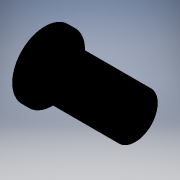
# Autodesk Inventor part: HFROLL5_a
Saved by Autodesk Inventor 2017.3 (Build 213256000, 256)
## iProperties
Part Number: HFROLL5_a
Material: Generic
Catalog Web Link: www.cadenas.de
Description: HFROLL, HFROLLM_ac-Rollers for Aluminum Frames
Vendor: MISUMI
Document SubType Name: Modeling
Designer: partserver
Manufacturer: MISUMI
Mass: 0.70535 g
Surface Area: 10.8347 cm^2
Volume: 0.70535 cm^3
Density: 1 g/cm^3
Appearance: PSOLRGB-0-0-0
Category: PARTsolutions
Company: MISUMI
Title: HFROLL5
Author: Cadenas PARTsolutions
Comments: Rollers for Aluminum Frames
PSOL_IDENT_0: {$CADENAS_DATA\23d-libs\misumi\metric\39_accessories_for_al_extrusions\hfroll\hfroll_ac.prj},173 {VT
PSOL_IDENT_1: YP=3D},{NB=HFROLL5_a},{LINA=HFROLL5},{NN=HFROLL, HFROLLM_ac},{DATE=30.03.2018 07:06:35},{GEOMDATE=10
PSOL_IDENT_2: .06.2016 08:24:00},{VERSION=},{LINEID=10},{WBVAR=MATAC},{WBNUMERIC=}  {NB=HFROLL5_a},{LINA=HFROLL5},
PSOL_IDENT_3: {KT=DUMMY},{PN=HFROLL5},{MATAC=HFROLL},{MATR=Nylon 6},{TYPE=HFROLL},{NO=5},{CFSW=6},{CFT=20-40 Sq.},
PSOL_IDENT_4: {H=6.0},{D=24},{T=15.0},{TT1=4},{TT2=5},{DD1=29.0},{DD2=9.2},{COLOR=Black},{BEARING=None},{ACL=16.5}
PSOL_IDENT_5: ,{ACTT3=1.5},{ACD2=9},{ACDD4=6.2},{ACDD5=13},{QAC=1},{COL=0.00,0.00,0.00,0.00}
NB: HFROLL5_a
NN: HFROLL, HFROLLM_ac
NT: Rollers for Aluminum Frames
NBSYN: $PN._a
LINA: HFROLL5
CATALOG: Misumi
MATAC: Nylon 6
MATR: Nylon 6
NO: 5
CFSW: 6
CFT: 20-40 Sq.
H: 6
D: 24
T: 15
TT1: 4
TT2: 5
DD1: 29
DD2: 9.2
COLOR: Black
ACL: 16.5
ACTT3: 1.5
ACD2: 9
ACDD4: 6.2
ACDD5: 13
QAC: 1
SUPPLIER: MISUMI
ARTICLENO: HFROLL5_a
BOMINFO: HFROLL5
CREATOR: CADENAS GmbH
Autodesk Inventor part; units mm, degrees
sketch "Sketch_1" plane through (0, 0, 0) normal (0, 0, 1) x (1, 0, 0)
  line L0 (1.5, 0) -> (-16.5, 0)
  line L1 (-16.5, 4.5) -> (-16.5, 3.1)
  line L2 (-16.5, 3.1) -> (1.5, 3.1)
  line L3 (1.5, 3.1) -> (1.5, 6.5)
  line L4 (1.5, 6.5) -> (0, 6.5)
  line L5 (0, 6.5) -> (0, 4.5)
  line L6 (0, 4.5) -> (-16.5, 4.5)
  constraints: 14 end point
revolve "Revolution1" add sketch "Sketch_1" angle 360 about axis through (1.5, 0, 0) along (1, 0, 0)
ref_plane "to_roller_XY" through (0, 0, 0) normal (1, 0, 0) x (0, 0, -1)
ref_plane "to_roller_YZ" through (0, 0, 0) normal (0, 0, -1) x (0, 1, 0)
ref_plane "to_roller_ZX" through (0, 0, 0) normal (0, 1, 0) x (1, 0, 0)
body "Solid1"
